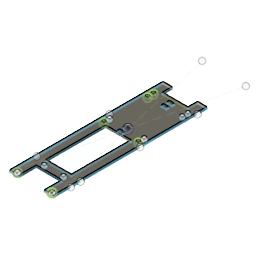
H Bracket (Autodesk Fusion 360 design; units mm, degrees)
part number: 2026-02-18-15-30-19-478
Autodesk Fusion 360 part; units mm, degrees
sketch "Sketch1" plane through (0, 0, 0) normal (0, 0, 1) x (1, 0, 0)
  line L0 (-22.75, 59.25) -> (-22.75, -100)
  line L1 (22.75, -100) -> (22.75, 59.25)
  line L2 (22.75, 100) -> (-22.75, -100) construction
  line L3 (-22.75, 100) -> (22.75, -100) construction
  circle A0 centre (-18, -97) radius 1.75
  circle A1 centre (18, -97) radius 1.75
  line L4 (-22.75, -100) -> (-13.25, -100)
  line L5 (-22.75, 59.25) -> (-22.75, -100)
  line L6 (13.25, -100) -> (22.75, -100)
  line L7 (22.75, -100) -> (22.75, 59.25)
  line L8 (22.75, -82) -> (22.75, -72)
  line L9 (-22.75, -72) -> (-22.75, -82)
  circle A2 centre (-10, -77) radius 1.75
  circle A3 centre (10, -77) radius 1.75
  circle A4 centre (-18, -97) radius 1.75
  circle A5 centre (18, -97) radius 1.75
  circle A6 centre (-18, -7) radius 1.75
  circle A7 centre (18, -7) radius 1.75
  line L10 (-13.25, -10) -> (13.25, -10)
  line L11 (22.75, -10) -> (22.75, 3.5531)
  line L12 (-22.75, 3.5531) -> (-22.75, -10)
  circle A8 centre (-18, 38.5) radius 1.75
  circle A9 centre (18, 38.5) radius 1.75
  circle A10 centre (-18, -1) radius 1.75
  circle A11 centre (18, -1) radius 1.75
  circle A12 centre (-18, 44.5) radius 1.75
  circle A13 centre (18, 44.5) radius 1.75
  line L13 (0.8083, 3.5531) -> (-0.8083, 3.5531)
  line L14 (-22.75, -100) -> (-13.25, -100)
  line L15 (13.25, -100) -> (22.75, -100)
  line L16 (13.25, 59.25) -> (13.25, 49.5)
  line L17 (-13.25, 49.5) -> (-13.25, 59.25)
  line L18 (-13.25, -82) -> (13.25, -82)
  line L19 (13.25, -72) -> (-13.25, -72)
  line L20 (-13.25, -100) -> (-13.25, -82)
  line L21 (-13.25, -72) -> (-13.25, -10)
  line L22 (13.25, -10) -> (13.25, -72)
  line L23 (13.25, -82) -> (13.25, -100)
  line L24 (22.75, 49.5) -> (23, 49.5)
  line L25 (-13.25, 49.25) -> (13.25, 49.25)
  line L26 (-13.25, 49.5) -> (-13.25, 49.25)
  line L27 (13.25, 49.5) -> (13.25, 49.25)
  line L28 (-22.75, 59.25) -> (-13.25, 59.25)
  line L29 (13.25, 59.25) -> (22.75, 59.25)
  line L30 (2.5, 37.5) -> (-2.5, 37.5)
  line L31 (-2.5, 37.5) -> (-2.5, 39.5)
  line L32 (-2.5, 39.5) -> (2.5, 39.5)
  line L33 (2.5, 39.5) -> (2.5, 37.5)
  line L34 (2.5, 37.5) -> (-2.5, 39.5) construction
  line L35 (-2.5, 37.5) -> (2.5, 39.5) construction
  line L36 (-2.5, 45.5) -> (2.5, 45.5)
  line L37 (2.5, 45.5) -> (2.5, 43.5)
  line L38 (2.5, 43.5) -> (-2.5, 43.5)
  line L39 (-2.5, 43.5) -> (-2.5, 45.5)
  line L40 (-2.5, 45.5) -> (2.5, 43.5) construction
  line L41 (2.5, 45.5) -> (-2.5, 43.5) construction
  line L42 (-2.5, 0) -> (2.5, 0)
  line L43 (2.5, 0) -> (2.5, -2)
  line L44 (2.5, -2) -> (-2.5, -2)
  line L45 (-2.5, -2) -> (-2.5, 0)
  line L46 (-2.5, 0) -> (2.5, -2) construction
  line L47 (2.5, 0) -> (-2.5, -2) construction
  line L48 (-2.5, -6) -> (2.5, -6)
  line L49 (2.5, -6) -> (2.5, -8)
  line L50 (2.5, -8) -> (-2.5, -8)
  line L51 (-2.5, -8) -> (-2.5, -6)
  line L52 (-2.5, -6) -> (2.5, -8) construction
  line L53 (2.5, -6) -> (-2.5, -8) construction
  line L54 (-0.2275, -1) -> (0.2275, -1)
  dimension "d1" = 45.5
  dimension "d2" = 200
  dimension "d4" = 3.5
  dimension "d5" = 3.5
  dimension "d6" = 3
  dimension "d7" = 3
  dimension "d10" = 9.5
  dimension "d13" = 200
  dimension "d14" = 10
  dimension "d16" = 3.5
  dimension "d17" = 5
  dimension "d19" = 3.5
  dimension "d20" = 5
  dimension "d22" = 3.5
  dimension "d23" = 3.5
  dimension "d30" = 3.5
  dimension "d31" = 3.5
  dimension "d34" = 90
  dimension "d35" = 90
  dimension "d36" = 3
  dimension "d37" = 3.5
  dimension "d38" = 3.5
  dimension "d41" = 45.5
  dimension "d42" = 45.5
  dimension "d43" = 3.5
  dimension "d44" = 3.5
  dimension "d45" = 18
  dimension "d47" = 6
  dimension "d48" = 6
  dimension "d49" = 3.5
  dimension "d50" = 3.5
  dimension "d53" = 6
  dimension "d54" = 6
  dimension "d57" = 45.5
  dimension "d59" = 9.75
  dimension "d61" = 4.75
  dimension "d62" = 0.25
  dimension "d63" = 0.25
  dimension "d64" = 10
  dimension "d67" = 5
  dimension "d68" = 2
  dimension "d69" = 5
  dimension "d70" = 2
  dimension "d71" = 5
  dimension "d72" = 2
  dimension "d73" = 5
  dimension "d74" = 2
  constraint parallel L0 L1
  constraint coincident L2 origin
  constraint coincident L3 origin
  constraint horizontal L4
  constraint vertical L20
  constraint vertical L5
  constraint vertical L16
  constraint horizontal L6
  constraint vertical L7
  constraint vertical L8
  constraint vertical L9
  constraint coincident L0 L9.end
  constraint horizontal L10
  constraint vertical L11
  constraint vertical L12
  constraint coincident L1 L11.end
  constraint coincident L5 L12.end
  constraint coincident L2 L13.start
  constraint coincident L3 L13.end
  constraint collinear L14 L15
  constraint collinear L16 L22
  constraint collinear L17 L21
  constraint collinear L20 L21
  constraint collinear L22 L23
  constraint perpendicular L7 L29
  constraint perpendicular L16 L24
  constraint perpendicular L0 L25
  constraint vertical L27
  constraint coincident L1 L24.start
  constraint collinear L28 L29
  constraint horizontal L30
  constraint perpendicular L30 L31
  constraint parallel L30 L32
  constraint parallel L31 L33
  constraint horizontal L36
  constraint perpendicular L36 L37
  constraint parallel L36 L38
  constraint parallel L37 L39
  constraint horizontal L42
  constraint perpendicular L42 L43
  constraint parallel L42 L44
  constraint parallel L43 L45
  constraint horizontal L48
  constraint perpendicular L48 L49
  constraint parallel L48 L50
  constraint parallel L49 L51
  constraint coincident L3 L54.end
  constraint coincident L2 L54.start
  measures "d1" distance of L0.end L1.start
  measures "d2" distance of L3.start L0.end
  measures "d4" diameter of A0
  measures "d5" diameter of A1
  measures "d6" distance of A0.centre L14
  measures "d7" distance of A1.centre L15
  measures "d10" distance of L0.end L4.end
  measures "d13" distance of L2.start L1.start
  measures "d14" distance of L9.end L9.start
  measures "d16" diameter of A2 A3
  measures "d17" distance of A2.centre L18
  measures "d19" diameter of A3
  measures "d20" distance of A3.centre L18
  measures "d22" diameter of A4
  measures "d23" diameter of A5
  measures "d30" diameter of A6
  measures "d31" diameter of A7
  measures "d34" distance of A0.centre A6.centre
  measures "d35" distance of A1.centre A7.centre
  measures "d36" distance of A6.centre L10
  measures "d37" diameter of A8
  measures "d38" diameter of A9
  measures "d41" distance of A6.centre A8.centre
  measures "d42" distance of A7.centre A9.centre
  measures "d43" diameter of A10
  measures "d44" diameter of A11
  measures "d45" horizontal distance of origin A11.centre
  measures "d47" distance of A6.centre A10.centre
  measures "d48" distance of A7.centre A11.centre
  measures "d49" diameter of A12
  measures "d50" diameter of A13
  measures "d53" distance of A8.centre A12.centre
  measures "d54" distance of A9.centre A13.centre
  measures "d57" distance of L0.start L1.end
  measures "d59" distance of L16.end L24.end
  measures "d61" distance of A12.centre L25
  measures "d62" distance of L17.start L25.start
  measures "d63" distance of L16.end L25.end
  measures "d64" distance of L25 L28
  measures "d67" distance of L31.end L32.end L14
  measures "d68" distance of L30.end L31.end L14
  measures "d69" distance of L37.end L38.end
  measures "d70" distance of L36.end L37.end
  measures "d71" distance of L43.end L44.end
  measures "d72" distance of L42.end L43.end
  measures "d73" distance of L49.end L50.end
  measures "d74" distance of L48.end L49.end
extrude "Extrude1" add sketch "Sketch1" along normal blind 2 contours L0 L1 L4 L5 L6 L7 L8 L9 L11 L12 L14 L15 L16 L17 L18 L20 L23 L25 L26 L27 L28 L29 | L30 L31 L32 L33 | L36 L37 L38 L39 | L42 L43 L44 L45 | L48 L49 L50 L51 makes body 1
extrude "Extrude2" add sketch "Sketch1" along normal blind 2 separate body makes body 2
extrude "Extrude3" add sketch "Sketch1" along normal blind 2 separate body makes body 3
extrude "Extrude4" cut 1 faces at (5.6485, 12.6322, 2) along direction (0, 0, -1) blind 2 on bodies 1 bodies 1 2 3
extrude "Extrude5" add sketch "Sketch1" along normal blind 2 bodies 1 2 3
